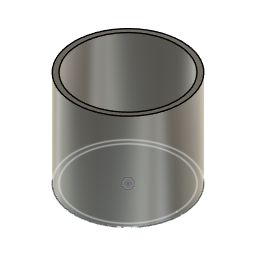
m07-m03 lens coupler v2 (Autodesk Fusion 360 design; units mm, degrees)
Autodesk Fusion 360 part; units mm, degrees
sketch "Sketch1" plane through (0, 0, 0) normal (0, 0, 1) x (1, 0, 0)
  circle A0 centre (0, 0) radius 15.2
  circle A1 centre (0, 0) radius 16.7
  dimension "d1" = 30.4
  dimension "d2" = 1.5
  constraint coincident A0.centre A1.centre
  measures "d1" diameter of A0
extrude "Extrude1" add sketch "Sketch1" along normal blind 30
